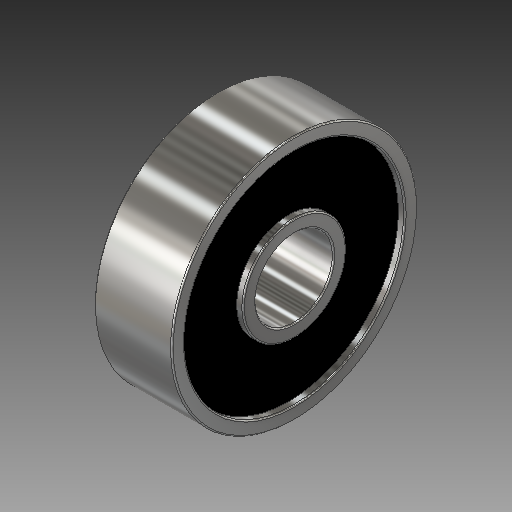
# Autodesk Inventor part: Подшипник 685
Saved by Autodesk Inventor 2018 (Build 220112000, 112)
## iProperties
Part Number: Подшипник 685
Material: Типовые
Document SubType Name: Modeling
Designer: sbnnl
Density: 1 g/cm^3
Appearance: Хром - полированный
Author: sbnnl
Autodesk Inventor part; units mm, degrees
ref_plane "YZ Plane" through (0, 0, 0) normal (1, 0, 0) x (0, 1, 0)
ref_plane "XZ Plane" through (0, 0, 0) normal (0, 1, 0) x (-1, 0, 0)
ref_plane "XY Plane" through (0, 0, 0) normal (0, 0, 1) x (1, 0, 0)
sketch "Эскиз1" plane through (0, 0, 0) normal (1, 0, 0) x (0, 1, 0)
  circle A0 centre (0, 0) radius 3
  circle A1 centre (0, 0) radius 9.5
  dimension "d0" = 6
  dimension "d1" = 19
  constraints: 2 centre point, 2 coincident
  measures "d0" diameter of A0
  measures "d1" diameter of A1
extrude "Выдавливание1" add sketch "Эскиз1" along normal blind 6
sketch "Эскиз2" plane through (6, 0, 0) normal (1, 0, 0) x (0, 0, -1)
  circle A0 centre (0, 0) radius 4
  circle A1 centre (0, 0) radius 8.5
  dimension "d4" = 8
  dimension "d5" = 17
  constraints: 2 centre point, 2 coincident
  measures "d4" diameter of A0
  measures "d5" diameter of A1
extrude "Выдавливание2" cut sketch "Эскиз2" against normal blind 0.5
sketch "Эскиз3" plane through (0, 0, 0) normal (-1, 0, 0) x (0, 0, 1)
  circle A0 centre (0, 0) radius 4 projected
  circle A1 centre (0, 0) radius 8.5 projected
  circle A2 centre (0, 0) radius 4
  circle A3 centre (0, 0) radius 8.5
  constraints: 2 centre point, 2 coincident, 2 concentric
extrude "Выдавливание3" cut sketch "Эскиз3" against normal blind 0.5
fillet "Сопряжение1" radius 0.1 8 edges at (6, -9.5, 0) (6, 0, 8.5) (6, 0, 4) (6, -3, 0) (0, -9.5, 0) (0, 0, -8.5) (0, 0, -4) (0, -3, 0)
